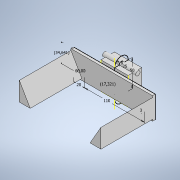
# Autodesk Inventor part: Doigt trans
Saved by Autodesk Inventor 2022 (Build 260153000, 153)
## iProperties
Created: 2022-04-26
Part Number: Doigt trans
Material: Générique
Document SubType Name: Modeling
Designer: victo
Density: 1 g/cm^3
Appearance: Par défaut
Author: victo
Autodesk Inventor part; units mm, degrees
ref_plane "YZ Plane" through (0, 0, 0) normal (1, 0, 0) x (0, 1, 0)
ref_plane "XZ Plane" through (0, 0, 0) normal (0, 1, 0) x (-1, 0, 0)
ref_plane "XY Plane" through (0, 0, 0) normal (0, 0, 1) x (1, 0, 0)
sketch "Esquisse1" plane through (0, 0, 0) normal (1, 0, 0) x (0, 1, 0)
  line L0 (25, -12.5) -> (-25, -12.5)
  line L1 (-25, -12.5) -> (-25, 12.5)
  line L2 (-25, 12.5) -> (25, 12.5)
  line L3 (25, 12.5) -> (25, -12.5)
  line L4 (25, -12.5) -> (-25, 12.5) construction
  line L5 (-25, -12.5) -> (25, 12.5) construction
  circle A0 centre (25, 0) radius 12.5
  circle A1 centre (25, 0) radius 4
  circle A2 centre (-25, 0) radius 4
  circle A3 centre (-25, 0) radius 12.5
  point P0 (0, 0)
  point P1 (-25, -12.5)
  point P2 (25, -12.5)
  point P3 (25, -4)
  point P4 (25, 4)
  point P5 (-25, 4)
  point P6 (-25, -4)
  dimension "d1" = 25
  dimension "d0" = 8
  dimension "d2" = 50
  constraints: 12 end point, 4 midpoint, 2 centre point, 2 coincident, 2 parallel, 1 equal radius, 1 horizontal, 1 perpendicular, 6 other
  measures "d0" diameter of A1
  measures "d2" distance between parallel lines of L3 L1
extrude "Extrusion1" add sketch "Esquisse1" along normal mid plane 61 contours A1 L3 | L3 A1 | A2 L1 | L1 A2
extrude "Extrusion2" add sketch "Esquisse1" along normal mid plane 50 contours A0 L3 A1 | L0 A3 L2 A0 | L1 A2 A3 picked at (24.0029, -9.5456) picked at (-15.4378, -0.9272)
sketch "Esquisse2" plane through (-25, -25, 12.5) normal (0, 0, 1) x (1, 0, 0)
  line L0 (0, 0) -> (0, 50) projected
  line L1 (50, 50) -> (50, 0) projected
  line L2 (0, 0) -> (50, 0) projected
  line L3 (-50, 7.6795) -> (-30, 7.6795)
  line L4 (-30, 7.6795) -> (25, 7.6795)
  line L5 (25, 7.6795) -> (80, 7.6795)
  line L6 (80, 7.6795) -> (100, 7.6795)
  line L7 (100, 7.6795) -> (100, 42.3205)
  line L8 (100, 42.3205) -> (80, 7.6795)
  line L9 (-30, 7.6795) -> (-50, 42.3205)
  line L10 (-50, 42.3205) -> (-50, 7.6795)
  line L11 (25, -15.6) -> (25, 65.6) projected
  line L12 (-50, 45.3205) -> (100, 45.3205)
  line L13 (100, 45.3205) -> (100, 4.6795)
  line L14 (100, 4.6795) -> (-50, 4.6795)
  line L15 (-50, 4.6795) -> (-50, 45.3205)
  line L16 (-50, 42.3205) -> (-50, 45.3205) construction
  line L17 (-50, 7.6795) -> (-50, 4.6795) construction
  line L18 (100, 42.3205) -> (100, 45.3205) construction
  line L19 (100, 7.6795) -> (100, 4.6795) construction
  line L20 (-50, 4.6795) -> (25, 25) construction
  line L21 (25, 25) -> (100, 45.3205) construction
  dimension "d14" = 34.641
  dimension "d15" = 110
  dimension "d16" = 20
  dimension "d17" = 17.3205
  dimension "d18" = 60
  dimension "d22" = 3
  constraints: 36 end point, 7 equal length, 4 point on line, 3 perpendicular, 2 horizontal, 2 parallel, 1 collinear
  measures "d14" distance of L9.end L3.start
  measures "d15" distance of L5.end L3.end
  measures "d16" distance of L3.start L3.end
  measures "d17" distance of L20.end L4.end
  measures "d18" angle of L9 L3
  measures "d22" distance between parallel lines of L5 L14
extrude "Extrusion3" add sketch "Esquisse2" along normal blind 100 contours L3 L10 L9 | L8 L7 L6
extrude "Extrusion4" add sketch "Esquisse2" along normal blind 5 contours L14 L15 L3 L4 L0 | L0 L4 L11 L14 | L4 L9 L15 L12 L0 | L0 L12 L11 L4 | L11 L5 L1 L14 | L3 L10 L9 | L11 L12 L1 L5 | L1 L5 L6 L13 L14 | L1 L12 L13 L8 L5 | L8 L7 L6
